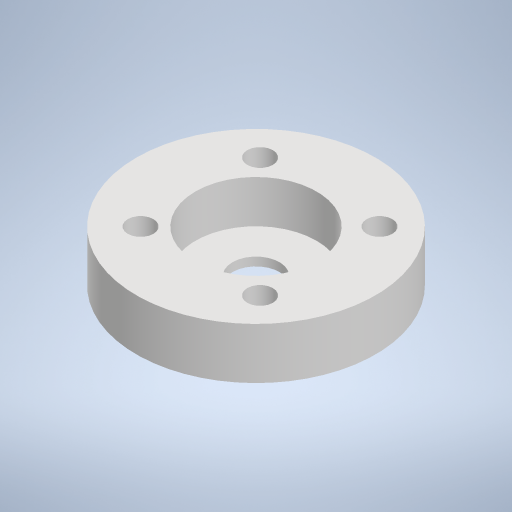
# Autodesk Inventor part: rhtgt; gjlibgybrf
Saved by Autodesk Inventor 2024.2 (Build 282272000, 272)
## iProperties
Created: 2026-03-15
Part Number: rhtgt; gjlibgybrf
Material: Типовые
Document SubType Name: Modeling
Designer: Service
Density: 1 g/cm^3
Appearance: По умолчанию
Author: Service
Autodesk Inventor part; units mm, degrees
ref_plane "YZ Plane" through (0, 0, 0) normal (1, 0, 0) x (0, 1, 0)
ref_plane "XZ Plane" through (0, 0, 0) normal (0, 1, 0) x (-1, 0, 0)
ref_plane "XY Plane" through (0, 0, 0) normal (0, 0, 1) x (1, 0, 0)
sketch "Эскиз1" plane through (0, 0, 0) normal (0, 1, 0) x (-1, 0, 0)
  circle A0 centre (0, 0) radius 14
  circle A1 centre (0, 0) radius 7.1
  circle A2 centre (6.7581, 6.7661) radius 1.5 projected
  circle A3 centre (-7.2419, -7.2339) radius 1.5 projected
  circle A4 centre (-7.2419, 6.7661) radius 1.5 projected
  circle A5 centre (6.7581, -7.2339) radius 1.5 projected
  circle A6 centre (0, 0) radius 2.75
  dimension "d0" = 28
  dimension "d1" = 14.2
  dimension "d4" = 5.5
  constraints: 3 centre point, 3 coincident
  measures "d0" diameter of A0
  measures "d1" diameter of A1
  measures "d4" diameter of A6
extrude "Выдавливание2" add sketch "Эскиз1" along normal blind 6 contours A0
extrude "Выдавливание3" add sketch "Эскиз1" along normal blind 1 contours A1
sketch "Эскиз2" plane through (0, 0, 0) normal (0, -1, 0) x (1, 0, 0)
  line L0 (-9.0814, -5.0692) -> (-6.0451, -4.1396)
  line L1 (-6.0451, -4.1396) -> (-3.7219, -6.3042)
  line L2 (-3.7219, -6.3042) -> (-4.4349, -9.3986)
  line L3 (-4.4349, -9.3986) -> (-7.4712, -10.3282)
  line L4 (-7.4712, -10.3282) -> (-9.7944, -8.1636)
  line L5 (-9.7944, -8.1636) -> (-9.0814, -5.0692)
  circle A0 centre (-6.7581, -7.2339) radius 1.5 projected
  circle A1 centre (-6.7581, 6.7661) radius 1.5 projected
  circle A2 centre (7.2419, 6.7661) radius 1.5 projected
  circle A3 centre (7.2419, -7.2339) radius 1.5 projected
  line L6 (-9.0814, 8.9308) -> (-6.0451, 9.8604)
  line L7 (-6.0451, 9.8604) -> (-3.7219, 7.6958)
  line L8 (-3.7219, 7.6958) -> (-4.4349, 4.6014)
  line L9 (-4.4349, 4.6014) -> (-7.4712, 3.6718)
  line L10 (-7.4712, 3.6718) -> (-9.7944, 5.8364)
  line L11 (-9.7944, 5.8364) -> (-9.0814, 8.9308)
  line L12 (4.9186, 8.9308) -> (7.9549, 9.8604)
  line L13 (7.9549, 9.8604) -> (10.2781, 7.6958)
  line L14 (10.2781, 7.6958) -> (9.5651, 4.6014)
  line L15 (9.5651, 4.6014) -> (6.5288, 3.6718)
  line L16 (6.5288, 3.6718) -> (4.2056, 5.8364)
  line L17 (4.2056, 5.8364) -> (4.9186, 8.9308)
  line L18 (4.8052, -5.0148) -> (7.8414, -4.0851)
  line L19 (7.8414, -4.0851) -> (10.1647, -6.2498)
  line L20 (10.1647, -6.2498) -> (9.4517, -9.3441)
  line L21 (9.4517, -9.3441) -> (6.4154, -10.2738)
  line L22 (6.4154, -10.2738) -> (4.0921, -8.1091)
  line L23 (4.0921, -8.1091) -> (4.8052, -5.0148)
  line L24 (-9.0814, -5.0692) -> (-6.0451, -4.1396)
  line L25 (-6.0451, -4.1396) -> (-3.7219, -6.3042)
  line L26 (-3.7219, -6.3042) -> (-4.4349, -9.3986)
  line L27 (-4.4349, -9.3986) -> (-7.4712, -10.3282)
  line L28 (-7.4712, -10.3282) -> (-9.7944, -8.1636)
  line L29 (-9.7944, -8.1636) -> (-9.0814, -5.0692)
  point P0 (0, 0)
  dimension "d9" = 5.5
  dimension "d12" = 5.5
  dimension "d13" = 5.5
  dimension "d14" = 5.5
  dimension "d15" = 5.5
  constraints: 60 end point, 1 coincident, 13 other
  measures "d9" distance between parallel lines of L2 L5
  measures "d12" distance between parallel lines of L8 L11
  measures "d13" distance between parallel lines of L14 L17
  measures "d14" distance between parallel lines of L20 L23
  measures "d15" distance between parallel lines of L26 L29
extrude "Выдавливание4" cut sketch "Эскиз2" against normal blind 2.4 contours L0 L1 L2 L3 L4 L5 | A1 | L6 L7 L8 L9 L10 L11 | L12 L13 L14 L15 L16 L17 | L18 L19 L20 L21 L22 L23
